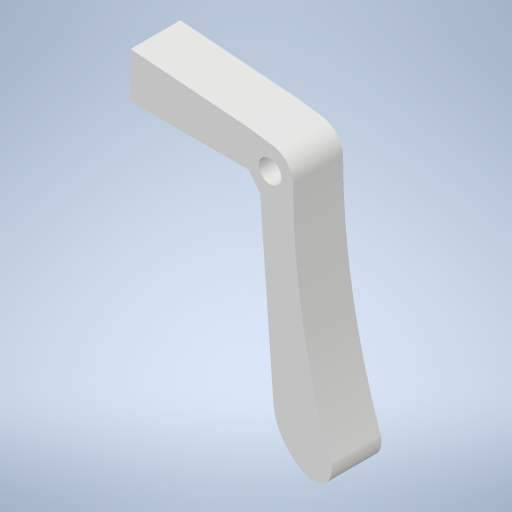
# Autodesk Inventor part: end_cap
Saved by Autodesk Inventor 2023 (Build 270158000, 158)
## iProperties
Created: 2026-02-12
Part Number: end_cap
Material: Типовые
Document SubType Name: Modeling
Designer: garin
Density: 1 g/cm^3
Appearance: По умолчанию
Author: garin
Autodesk Inventor part; units mm, degrees
ref_plane "YZ Plane" through (0, 0, 0) normal (1, 0, 0) x (0, 1, 0)
ref_plane "XZ Plane" through (0, 0, 0) normal (0, 1, 0) x (-1, 0, 0)
ref_plane "XY Plane" through (0, 0, 0) normal (0, 0, 1) x (1, 0, 0)
sketch "Эскиз3" plane through (0, 0, 0) normal (0, 0, 1) x (1, 0, 0)
  line L0 (0, 0) -> (0, -2.7467) construction
  line L1 (0, -2.7467) -> (11.9564, -2.7467) construction
  line L2 (11.9564, -2.7467) -> (9.408, -2.7467) construction
  line L3 (9.408, -2.7467) -> (9.408, -5.7467) construction
  line L4 (9.408, -5.7467) -> (11.9564, -5.7467) construction
  line L5 (11.9564, -5.7467) -> (11.9564, -2.7467) construction
  line L6 (0, -2.7467) -> (-5, -2.7467) construction
  circle A0 centre (9.408, -5.7467) radius 1.25
  circle A1 centre (9.408, -5.7467) radius 1.75
  line L7 (7, -2.7467) -> (8.3014, -4.391)
  line L8 (11.158, -5.7467) -> (11.9564, -5.7467)
  line L9 (7.0022, -6.7467) -> (8.3036, -8.3345)
  line L10 (8.3036, -8.3345) -> (9.7744, -27.7168)
  line L11 (15.7572, -33.2628) -> (17.1953, -33.2628)
  arc A2 (11.9564, -5.7467) -> (17.1953, -33.2628) centre (86.8368, -5.7467) ccw
  line L12 (-5.9978, -6.7467) -> (7.0022, -6.7467)
  arc A3 (9.7744, -27.7168) -> (15.7572, -33.2628) centre (15.7572, -27.2628) ccw
  line L13 (-5.9978, -6.7467) -> (-5.9978, -1.7467)
  line L14 (-5.9978, -1.7467) -> (7, -2.7467)
  line L15 (8.6118, -4.7831) -> (7.6809, -3.6069)
  line L16 (10.658, -5.7467) -> (11.9564, -5.7467)
  arc A4 (11.9564, -5.7467) -> (7.6809, -3.6069) centre (9.2832, -5.7467) ccw
  line L17 (7, -2.7467) -> (9.8806, -3.1411)
  point P0 (10.1953, -33.2628)
  point P1 (-5, -0.7467)
  point P2 (9.4081, -3.0764)
  dimension "d21" = 2.5
  dimension "d22" = 3.5
  dimension "d24" = 25
  dimension "d25" = 145
  dimension "d26" = 7
  dimension "d29" = 6
  dimension "d31" = 5
  dimension "d34" = 1.5
  constraints: 36 end point, 11 point on circle, 6 point on line, 5 centre point, 4 tangent, 3 coincident, 3 horizontal, 2 collinear, 2 parallel, 2 perpendicular, 2 vertical
  measures "d21" diameter of A0
  measures "d22" diameter of A1
  measures "d24" distance of L9.end point (10.195, -33.263)
  measures "d25" angle of L9 L10
  measures "d26" distance of point (10.195, -33.263) L11.end
  measures "d29" radius of A3
  measures "d31" distance of L12.start L13.end
  measures "d34" distance of L15.start L15.end
extrude "Выдавливание1" add sketch "Эскиз3" along normal blind 5.5 contours L16 A1 L15 A0 | A0 L15 A1 L16 | L8 A2 L11 A3 L10 L9 L12 L13 L14 L7 A1 | A1 L7 A4 L17 L8 | L7 L17 A4 | L17 A4
fillet "Сопряжение1" radius 2 1 edges at (17.1953, -33.2628, 2.75)
